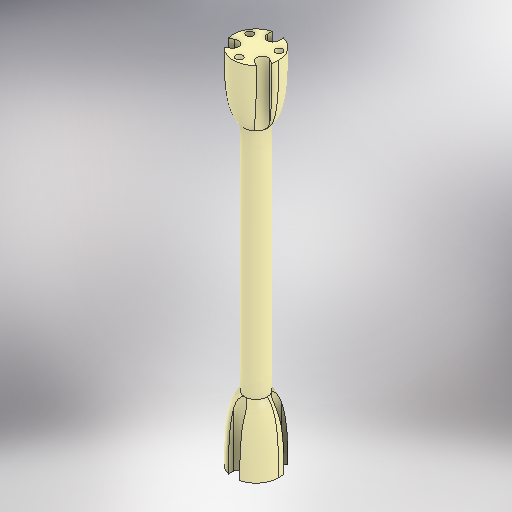
# Autodesk Inventor part: 8inch_spacer
Saved by Autodesk Inventor 2026 (Build 300175050, 175E)
## iProperties
Created: 2025-06-04
Part Number: 8inch_spacer
Material: Generic
Document SubType Name: Modeling
Designer: satom
Density: 1 g/cm^3
Appearance: Default
Author: satom
Autodesk Inventor part; units mm, degrees
ref_plane "YZ Plane" through (0, 0, 0) normal (1, 0, 0) x (0, 1, 0)
ref_plane "XZ Plane" through (0, 0, 0) normal (0, 1, 0) x (-1, 0, 0)
ref_plane "XY Plane" through (0, 0, 0) normal (0, 0, 1) x (1, 0, 0)
sketch "Sketch1" plane through (0, 0, 0) normal (0, 0, 1) x (1, 0, 0)
  line L0 (0, -63.5) -> (0, -101.6)
  line L1 (0, -101.6) -> (12.7, -101.6)
  line L2 (0, -63.5) -> (8.7521, -63.02) construction
  line L3 (12.7, -89.3688) -> (12.7, -101.6) construction
  spline S0 degree 4 poles (0, -63.5) (8.7521, -63.02) (12.7, -69.8272) (12.7, -89.3688) (12.7, -101.6) knots 1 1 1 1 1 2 2 2 2 2
  line L4 (8.7521, -63.02) -> (12.7, -69.8272) construction
  line L5 (12.7, -69.8272) -> (12.7, -89.3688) construction
  line L6 (-41.8785, 0) -> (51.4087, 0)
  line L7 (0, 63.5) -> (0, 101.6)
  line L8 (0, 101.6) -> (12.7, 101.6)
  line L9 (0, 63.5) -> (8.7521, 63.02) construction
  line L10 (12.7, 89.3688) -> (12.7, 101.6) construction
  spline S1 degree 4 poles (0, 63.5) (8.7521, 63.02) (12.7, 69.8272) (12.7, 89.3688) (12.7, 101.6) knots 1 1 1 1 1 2 2 2 2 2
  line L11 (8.7521, 63.02) -> (12.7, 69.8272) construction
  line L12 (12.7, 69.8272) -> (12.7, 89.3688) construction
  point P0 (0, 0)
  dimension "d2" = 38.1
  dimension "d3" = 12.7
  dimension "d5" = 101.6
  dimension "d50" = 63.02
  dimension "d51" = 69.8272
  dimension "d52" = 89.3688
  constraints: 10 end point, 6 symmetric about line, 1 horizontal, 1 perpendicular, 1 vertical, 6 other
  measures "d2" distance of L0.start L0.end
  measures "d3" distance of L0.end L1.end
  measures "d5" distance from line of L1 point (0, 0)
  measures "d50" vertical distance of L2.end point (0, 0)
  measures "d51" vertical distance of L4.end point (0, 0)
  measures "d52" vertical distance of L3.start point (0, 0)
revolve "Revolution1" add sketch "Sketch1" angle 360 about axis through (0, 63.5, 0) along (0, 1, 0)
sketch "Sketch2" plane through (0, 101.6, 0) normal (0, 1, 0) x (1, 0, 0)
  circle A0 centre (0, 0) radius 6.35
  point P0 (0, 0)
  dimension "d7" = 12.7
  constraints: 1 centre point, 1 coincident
  measures "d7" diameter of A0
extrude "Extrusion1" add sketch "Sketch2" against normal blind 203.2
sketch "Sketch3" plane through (0, 101.6, 0) normal (0, 1, 0) x (1, 0, 0)
  circle A0 centre (0, -9.525) radius 2
  circle A1 centre (8.2489, 4.7625) radius 2
  circle A2 centre (-8.2489, 4.7625) radius 2
  point P0 (0, 0)
  dimension "d10" = 9.525
  dimension "d11" = 4
  dimension "d14" = 360
  constraints: 3 centre point, 7 other
  measures "d10" distance of point (0, 0) A0.centre
  measures "d11" diameter of A0
extrude "Extrusion2" cut sketch "Sketch3" against normal blind 7
sketch "Sketch4" plane through (0, 101.6, 0) normal (0, 1, 0) x (1, 0, 0)
  line L0 (0, 9.525) -> (0, 15.875) construction
  line L1 (3.175, 9.525) -> (3.175, 15.875)
  line L2 (-3.175, 15.875) -> (-3.175, 9.525)
  arc A0 (-3.175, 9.525) -> (3.175, 9.525) centre (0, 9.525) ccw
  arc A1 (3.175, 15.875) -> (-3.175, 15.875) centre (0, 15.875) ccw
  line L3 (-9.8364, -2.0129) -> (-15.3357, -5.1879)
  line L4 (-12.1607, -10.6871) -> (-6.6614, -7.5121)
  arc A2 (-6.6614, -7.5121) -> (-9.8364, -2.0129) centre (-8.2489, -4.7625) ccw
  arc A3 (-15.3357, -5.1879) -> (-12.1607, -10.6871) centre (-13.7482, -7.9375) ccw
  line L5 (6.6614, -7.5121) -> (12.1607, -10.6871)
  line L6 (15.3357, -5.1879) -> (9.8364, -2.0129)
  arc A4 (9.8364, -2.0129) -> (6.6614, -7.5121) centre (8.2489, -4.7625) ccw
  arc A5 (12.1607, -10.6871) -> (15.3357, -5.1879) centre (13.7482, -7.9375) ccw
  point P0 (0, 0)
  point P1 (0, 12.7)
  point P2 (-10.9985, -6.35)
  point P3 (10.9985, -6.35)
  dimension "d18" = 9.525
  dimension "d19" = 3.175
  dimension "d20" = 6.35
  dimension "d23" = 360
  constraints: 16 end point, 12 point on circle, 6 centre point, 4 tangent, 1 midpoint, 1 parallel, 1 vertical, 34 other
  measures "d18" distance of point (0, 0) L0.start
  measures "d19" radius of A0
  measures "d20" distance of L0.start L0.end
extrude "Extrusion3" cut sketch "Sketch4" against normal blind 38.1
sketch "Sketch5" plane through (0, -101.6, 0) normal (0, -1, 0) x (1, 0, 0)
  circle A0 centre (0, -9.525) radius 2
  circle A1 centre (8.2489, 4.7625) radius 2
  circle A2 centre (-8.2489, 4.7625) radius 2
  point P0 (0, 0)
  dimension "d28" = 4
  dimension "d35" = 9.525
  dimension "d38" = 360
  constraints: 3 centre point, 7 other
  measures "d28" diameter of A0
  measures "d35" distance of A0.centre point (0, 0)
extrude "Extrusion4" cut sketch "Sketch5" against normal blind 7
sketch "Sketch6" plane through (0, -101.6, 0) normal (0, -1, 0) x (1, 0, 0)
  line L0 (0, 9.525) -> (0, 15.875) construction
  line L1 (3.175, 9.525) -> (3.175, 15.875)
  line L2 (-3.175, 15.875) -> (-3.175, 9.525)
  arc A0 (-3.175, 9.525) -> (3.175, 9.525) centre (0, 9.525) ccw
  arc A1 (3.175, 15.875) -> (-3.175, 15.875) centre (0, 15.875) ccw
  line L3 (-8.2489, -4.7625) -> (-13.7482, -7.9375) construction
  line L4 (-9.8364, -2.0129) -> (-15.3357, -5.1879)
  line L5 (-12.1607, -10.6871) -> (-6.6614, -7.5121)
  arc A2 (-6.6614, -7.5121) -> (-9.8364, -2.0129) centre (-8.2489, -4.7625) ccw
  arc A3 (-15.3357, -5.1879) -> (-12.1607, -10.6871) centre (-13.7482, -7.9375) ccw
  line L6 (8.2489, -4.7625) -> (13.7482, -7.9375) construction
  line L7 (6.6614, -7.5121) -> (12.1607, -10.6871)
  line L8 (15.3357, -5.1879) -> (9.8364, -2.0129)
  arc A4 (9.8364, -2.0129) -> (6.6614, -7.5121) centre (8.2489, -4.7625) ccw
  arc A5 (12.1607, -10.6871) -> (15.3357, -5.1879) centre (13.7482, -7.9375) ccw
  point P0 (0, 0)
  point P1 (0, 12.7)
  point P2 (-10.9985, -6.35)
  point P3 (10.9985, -6.35)
  dimension "d40" = 9.525
  dimension "d41" = 3.175
  dimension "d42" = 6.35
  dimension "d45" = 360
  constraints: 24 end point, 12 point on circle, 6 centre point, 4 tangent, 1 midpoint, 1 parallel, 1 vertical, 37 other
  measures "d40" distance of point (0, 0) L0.start
  measures "d41" radius of A0
  measures "d42" distance of L0.start L0.end
extrude "Extrusion5" cut sketch "Sketch6" against normal blind 38.1
body "Solid1"
